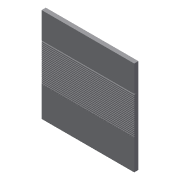
# Autodesk Inventor part: 00_chip_01_old
Saved by Autodesk Inventor 2019 (Build 230136000, 136)
## iProperties
Created: 2020-05-10
Part Number: 00_chip_01_old
Material: Generic
Document SubType Name: Modeling
Designer: diederichbenedict
Density: 1 g/cm^3
Appearance: Default
Author: diederichbenedict
Autodesk Inventor part; units mm, degrees
ref_plane "YZ Plane" through (0, 0, 0) normal (1, 0, 0) x (0, 1, 0)
ref_plane "XZ Plane" through (0, 0, 0) normal (0, 1, 0) x (-1, 0, 0)
ref_plane "XY Plane" through (0, 0, 0) normal (0, 0, 1) x (1, 0, 0)
sketch "Sketch1" plane through (0, 0, 0) normal (0, 0, 1) x (1, 0, 0)
  line L0 (0, 0) -> (23, 0)
  line L1 (23, 0) -> (23, 22.4)
  line L2 (23, 22.4) -> (0, 22.4)
  line L3 (0, 22.4) -> (0, 0)
  dimension "d0" = 23
  dimension "d1" = 22.4
  constraints: 8 end point, 2 parallel, 1 horizontal, 1 perpendicular
  measures "d0" distance of L2.end L1.end
  measures "d1" distance of L1.end L0.end
extrude "Extrusion1" add sketch "Sketch1" along normal blind 1
sketch "Sketch2" plane through (0, 0, 1) normal (0, 0, 1) x (1, 0, 0)
  line L0 (0, 0) -> (23, 0) projected
  line L1 (23, 0) -> (23, 22.4) projected
  line L2 (23, 22.4) -> (0, 22.4) projected
  line L3 (0, 22.4) -> (0, 0) projected
  line L4 (23, 0) -> (23, 22.4) projected
  line L5 (0, 16.13) -> (23, 16.13)
  line L6 (23, 16.13) -> (23, 7.13)
  line L7 (23, 7.13) -> (0, 7.13)
  line L8 (0, 7.13) -> (0, 16.13)
  dimension "d4" = 9
  dimension "d5" = 6.27
  constraints: 8 end point, 2 parallel, 2 point on line, 1 horizontal, 1 perpendicular
  measures "d4" distance of L5.end L6.end
  measures "d5" distance between parallel lines of L5 L2
extrude "Extrusion2" cut sketch "Sketch2" against normal blind 0.6 contours L3 L5 L1 L7
sketch "Sketch3" plane through (23, 0, 0) normal (1, 0, 0) x (0, 0, -1)
  line L0 (-1, 0) -> (-1, 7.13) projected
  line L1 (0, 0) -> (-1, 0) projected
  line L2 (0, 0) -> (0, 22.4) projected
  line L3 (0, 22.4) -> (-1, 22.4) projected
  circle A0 centre (-0.7, 15.7925) radius 0.3
  line L4 (-0.4, 16.13) -> (-0.4, 7.13) projected
  line L5 (-0.4, 7.13) -> (-1, 7.13) projected
  line L6 (-1, 16.13) -> (-1, 22.4) projected
  line L7 (-1, 16.13) -> (-0.4, 16.13) projected
  line L8 (-0.4, 16.13) -> (-0.4, 7.13) projected
  constraints: 1 centre point, 1 tangent
extrude "Extrusion3" add sketch "Sketch3" against normal up to surface (23 mm away) contours A0
pattern_linear "Rectangular Pattern1" count 24 spacing 0.39 along (0, -1, 0) of "Extrusion3"
sketch "Sketch4" plane through (0, 0, 1) normal (0, 0, 1) x (1, 0, 0)
  line L0 (0, 7.13) -> (0, 0) projected
  line L1 (0, 0) -> (23, 0) projected
  line L2 (23, 0) -> (23, 7.13) projected
  line L3 (23, 7.13) -> (0, 7.13) projected
  line L4 (23, 22.4) -> (22, 0)
  line L5 (0, 0) -> (23, 0) projected
  line L6 (22, 0) -> (23, 0)
  line L7 (23, 16.13) -> (23, 22.4) projected
  line L8 (23, 0) -> (23, 22.4)
  dimension "d16" = 1
  constraints: 6 end point, 2 perpendicular, 1 point on line
  measures "d16" distance of L4.end L1.end
extrude "Extrusion4" cut sketch "Sketch4" along normal through all both and the other way through all contours L4 L7 L8 L3 | L3 L2 L1 L4
body "Solid1"
